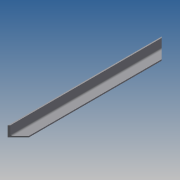
# Autodesk Inventor part: hubRingJigOuter
Saved by Autodesk Inventor 2014 SP1 (Build 180222100, 222)
## iProperties
Created: 2014-12-02
Part Number: hubRingJigOuter
Material: Generic
Document SubType Name: Modeling
Designer: Dave
Density: 1 g/cm^3
Appearance: Default
Author: Dave
Autodesk Inventor part; units mm, degrees
ref_plane "YZ Plane" through (0, 0, 0) normal (1, 0, 0) x (0, 1, 0)
ref_plane "XZ Plane" through (0, 0, 0) normal (0, 1, 0) x (-1, 0, 0)
ref_plane "XY Plane" through (0, 0, 0) normal (0, 0, 1) x (1, 0, 0)
sketch "Sketch1" plane through (0, 0, 0) normal (0, 0, 1) x (1, 0, 0)
  line L0 (0, 0) -> (0, 25.4)
  line L1 (0, 0) -> (25.4, 0)
  line L2 (3, 25.4) -> (3, 6.75)
  line L3 (6.75, 3) -> (25.4, 3)
  arc A0 (3, 6.75) -> (6.75, 3) centre (6.75, 6.75) ccw
  line L4 (0, 25.4) -> (3, 25.4)
  line L5 (25.4, 3) -> (25.4, 0)
  dimension "d0" = 25.4
  dimension "d1" = 25.4
  dimension "d2" = 3
  dimension "d3" = 3.75
  constraints: 12 end point, 3 perpendicular, 2 point on circle, 2 tangent, 1 centre point, 1 parallel, 1 vertical, 1 other
  measures "d0" distance of L0.start L0.end
  measures "d1" distance of L0.start L1.end
  measures "d2" distance between parallel lines of L2 L0
  measures "d3" radius of A0
extrude "Extrusion1" add sketch "Sketch1" along normal blind 373.38
sketch "Sketch10" plane through (0, 0, 0) normal (0, -1, 0) x (1, 0, 0)
  line L0 (25.4, 0) -> (0, 0) projected
  line L1 (25.4, 0) -> (25.4, 373.38) projected
  line L2 (0, 373.38) -> (25.4, 373.38) projected
  line L3 (0, 373.38) -> (25.4, 347.98)
  line L4 (0, 373.38) -> (70.5746, 373.38) construction
  line L5 (0, 0) -> (25.4, 25.4)
  line L6 (0, 0) -> (99.8075, 0) construction
  dimension "d36" = 45
  dimension "d37" = 45
  constraints: 8 end point, 2 horizontal, 2 point on line
  measures "d36" angle of L3 L4
  measures "d37" angle of L6 L5
extrude "Extrusion8" cut sketch "Sketch10" against normal blind 50.8
equation "\"d0\" = hubAngleWidth1"
equation "\"d1\" = hubAngleWidth2"
equation "\"d2\" = hubAngleThickness"
equation "\"d3\" = 1.25 * hubAngleThickness"
equation "\"hubAngleThickness\" = 3"
equation "\"hubAngleWidth1\" = 25.4"
equation "\"hubAngleWidth2\" = 25.4"
equation "\"hubCentralHoleOffset\" = 12.7"
body "Solid1"
